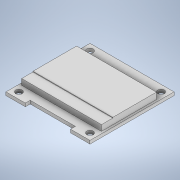
# Autodesk Inventor part: OLED Display
Saved by Autodesk Inventor 2022 (Build 260153000, 153)
## iProperties
Created: 2022-05-23
Part Number: OLED Display
Material: 일반
Document SubType Name: Modeling
Designer: user
Density: 1 g/cm^3
Appearance: 기본값
Author: user
Autodesk Inventor part; units mm, degrees
ref_plane "YZ Plane" through (0, 0, 0) normal (1, 0, 0) x (0, 1, 0)
ref_plane "XZ Plane" through (0, 0, 0) normal (0, 1, 0) x (-1, 0, 0)
ref_plane "XY Plane" through (0, 0, 0) normal (0, 0, 1) x (1, 0, 0)
sketch "스케치1" plane through (0, 0, 0) normal (0, 1, 0) x (-1, 0, 0)
  line L0 (-13, 13) -> (13, 13)
  line L1 (13, 13) -> (13, -13)
  line L2 (13, -13) -> (-13, -13)
  line L3 (-13, -13) -> (-13, 13)
  line L4 (-13, 13) -> (13, -13) construction
  line L5 (13, 13) -> (-13, -13) construction
  circle A0 centre (11, 11) radius 1
  line L6 (12.35, -8.2) -> (-12.35, -8.2)
  line L7 (-12.35, -8.2) -> (-12.35, 8.8)
  line L8 (-12.35, 8.8) -> (12.35, 8.8)
  line L9 (12.35, 8.8) -> (12.35, -8.2)
  line L10 (12.35, 5.3) -> (-12.35, 5.3)
  line L11 (0, 0) -> (0, -5.5368) construction
  line L12 (0, 0) -> (-4.847, 0) construction
  circle A1 centre (-11, 11) radius 1
  circle A2 centre (11, -11) radius 1
  circle A3 centre (-11, -11) radius 1
  dimension "d0" = 26
  dimension "d1" = 26
  dimension "d5" = 2
  dimension "d6" = 2
  dimension "d14" = 2
  dimension "d15" = 24.7
  dimension "d16" = 17
  dimension "d17" = 4.8
  dimension "d18" = 13.5
  constraints: 26 end point, 4 centre point, 4 parallel, 3 horizontal, 3 perpendicular, 3 symmetric about line, 2 midpoint, 2 point on line, 1 vertical, 3 other
  measures "d0" distance of L1.end L2.end
  measures "d1" distance of L0.end L1.end
  measures "d5" diameter of A0
  measures "d6" distance from line of L0 A0.centre
  measures "d14" distance from line of L1 A0.centre
  measures "d15" distance of L7.end L8.end
  measures "d16" distance of L6.end L7.end
  measures "d17" distance between parallel lines of L2 L6
  measures "d18" distance between parallel lines of L6 L10
extrude "돌출1" add sketch "스케치1" against normal blind 1 contours L0 L1 L2 L3 | L6 L7 L10 L9 | L10 L7 L8 L9
extrude "돌출3" add sketch "스케치1" along normal blind 2 contours L6 L7 L10 L9
extrude "돌출4" add sketch "스케치1" along normal blind 1.8 contours L10 L7 L8 L9
sketch "스케치2" plane through (0, 0, 0) normal (0, 1, 0) x (1, 0, 0)
  line L0 (-7, -11.5) -> (7, -11.5)
  line L1 (7, -11.5) -> (7, -14.5)
  line L2 (7, -14.5) -> (-7, -14.5)
  line L3 (-7, -14.5) -> (-7, -11.5)
  line L4 (13, -13) -> (-13, -13) projected
  line L5 (-7, -11.5) -> (7, -14.5) construction
  line L6 (7, -11.5) -> (-7, -14.5) construction
  point P0 (0, 0)
  point P1 (0, -13)
  dimension "d23" = 14
  dimension "d24" = 3
  constraints: 12 end point, 3 midpoint, 2 parallel, 1 horizontal, 1 perpendicular
  measures "d23" distance of L1.end L2.end
  measures "d24" distance of L0.end L1.end
extrude "돌출5" cut sketch "스케치2" against normal blind 16.75
